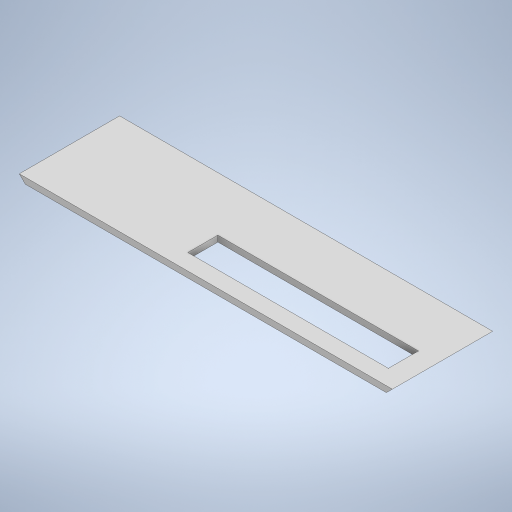
# Autodesk Inventor part: Back Wall
Saved by Autodesk Inventor 2023 (Build 270158000, 158)
## iProperties
Created: 2023-02-06
Part Number: Back Wall
Material: Generic
Document SubType Name: Modeling
Designer: Ahmed Nazir
Density: 1 g/cm^3
Appearance: Default
Author: Ahmed Nazir
Autodesk Inventor part; units mm, degrees
ref_plane "YZ Plane" through (0, 0, 0) normal (1, 0, 0) x (0, 1, 0)
ref_plane "XZ Plane" through (0, 0, 0) normal (0, 1, 0) x (-1, 0, 0)
ref_plane "XY Plane" through (0, 0, 0) normal (0, 0, 1) x (1, 0, 0)
sketch "Sketch1" plane through (0, 0, 0) normal (0, 1, 0) x (-1, 0, 0)
  line L0 (93, -25) -> (-93, -25)
  line L1 (-93, -25) -> (-93, 25)
  line L2 (-93, 25) -> (93, 25)
  line L3 (93, 25) -> (93, -25)
  line L4 (93, -25) -> (-93, 25) construction
  line L5 (-93, -25) -> (93, 25) construction
  line L6 (17, 2) -> (-83, 2)
  line L7 (-83, 2) -> (-83, 17)
  line L8 (-83, 17) -> (17, 17)
  line L9 (17, 17) -> (17, 2)
  point P0 (0, 0)
  point P1 (-83, 9.5)
  point P2 (-33, 17)
  dimension "d0" = 186
  dimension "d1" = 50
  dimension "d20" = 10
  dimension "d21" = 100
  dimension "d23" = 23
  dimension "d24" = 8
  constraints: 20 end point, 4 midpoint, 4 parallel, 2 horizontal, 2 perpendicular
  measures "d0" distance of L1.end L2.end
  measures "d1" distance of L0.end L1.end
  measures "d20" distance from line of L1 point (-83, 9.5)
  measures "d21" distance of L6.start L6.end
  measures "d23" distance between parallel lines of L2 L6
  measures "d24" distance between parallel lines of L8 L2
extrude "Extrusion1" add sketch "Sketch1" along normal blind 3
chamfer "Chamfer3" distance 3 angle 45 1 edges at (-93, 0, 0) measured on face at (-93, 1, -8.3333)
chamfer "Chamfer4" distance 3 angle 45 1 edges at (93, 0, 0) measured on face at (93, 1, 8.3333)
body "Solid1"
